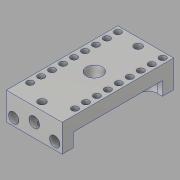
# Autodesk Inventor part: PocketNC_Vise_part2
Saved by Autodesk Inventor 2017 (Build 210142000, 142)
## iProperties
Created: 2018-06-05
Part Number: PocketNC_Vise_part2
Material: Aluminum 6061
Document SubType Name: Modeling
Designer: Jarrett
Density: 2.7 g/cm^3
Appearance: Aluminum - Flat
Author: Jarrett
Autodesk Inventor part; units mm, degrees
ref_plane "YZ Plane" through (0, 0, 0) normal (1, 0, 0) x (0, 1, 0)
ref_plane "XZ Plane" through (0, 0, 0) normal (0, 1, 0) x (-1, 0, 0)
ref_plane "XY Plane" through (0, 0, 0) normal (0, 0, 1) x (1, 0, 0)
sketch "Sketch1" plane through (0, 0, 0) normal (0, 1, 0) x (-1, 0, 0)
  line L0 (0, 0) -> (12.71, 0) construction
  line L1 (12.71, 25.41) -> (-12.71, 25.41)
  line L2 (-12.71, 25.41) -> (-12.71, -25.41)
  line L3 (-12.71, -25.41) -> (12.71, -25.41)
  line L4 (12.71, 25.41) -> (12.71, -25.41)
  dimension "d0" = 12.71
  dimension "d1" = 25.41
  dimension "d2" = 25.42
  dimension "d3" = 50.82
  constraints: 10 end point, 2 vertical, 1 horizontal, 1 perpendicular
  measures "d0" distance of L0.start L0.end
  measures "d1" distance of L0.end L1.start
  measures "d2" distance of L1.start L1.end
  measures "d3" distance of L1.end L2.end
extrude "Extrusion1" add sketch "Sketch1" along normal mid plane 12.6
sketch "Sketch2" plane through (0, -6.3, 0) normal (0, -1, 0) x (1, 0, 0)
  line L0 (12.71, 25.41) -> (12.71, 20.31) construction
  line L1 (12.71, 20.31) -> (6.26, 20.31)
  line L2 (12.71, -25.41) -> (12.71, -20.31) construction
  line L3 (12.71, -20.31) -> (6.26, -20.31)
  line L4 (6.26, -20.31) -> (6.26, 20.31)
  line L5 (12.71, 20.31) -> (12.71, -20.31)
  line L6 (12.71, 25.41) -> (12.71, -25.41) projected
  line L7 (0, 25.41) -> (0, -25.41)
  line L8 (-12.71, 20.31) -> (-6.26, 20.31)
  line L9 (-12.71, -20.31) -> (-6.26, -20.31)
  line L10 (-6.26, -20.31) -> (-6.26, 20.31)
  line L11 (-12.71, 20.31) -> (-12.71, -20.31)
  point P0 (0, 0)
  dimension "d6" = 5.1
  dimension "d7" = 6.45
  dimension "d8" = 5.1
  dimension "d9" = 6.45
  constraints: 22 end point, 4 symmetric about line, 2 perpendicular, 1 collinear, 1 vertical
  measures "d6" distance of L0.start L0.end
  measures "d7" distance of L0.end L1.end
  measures "d8" distance of L2.start L2.end
  measures "d9" distance of L2.end L3.end
extrude "Extrusion2" cut sketch "Sketch2" against normal blind 6.25
fillet "Fillet1" radius 4 4 edges at (6.26, -3.175, 20.31) (6.26, -3.175, -20.31) (-6.26, -3.175, -20.31) (-6.26, -3.175, 20.31)
sketch "Sketch3" plane through (0, 6.3, 0) normal (0, 1, 0) x (1, 0, 0)
  line L0 (-12.71, 25.41) -> (-12.71, 22.91) construction
  line L1 (-12.71, 22.91) -> (-10.21, 22.91) construction
  circle A0 centre (-10.21, 22.91) radius 1.5
  circle A1 centre (-10.21, -17.09) radius 1.5
  circle A2 centre (-10.21, -12.09) radius 1.5
  circle A3 centre (-10.21, -7.09) radius 1.5
  circle A4 centre (-10.21, -2.09) radius 1.5
  circle A5 centre (-10.21, 2.91) radius 1.5
  circle A6 centre (-10.21, 7.91) radius 1.5
  circle A7 centre (-10.21, 12.91) radius 1.5
  circle A8 centre (-10.21, 17.91) radius 1.5
  circle A9 centre (10.21, 22.91) radius 1.5
  circle A10 centre (10.21, -17.09) radius 1.5
  circle A11 centre (10.21, -12.09) radius 1.5
  circle A12 centre (10.21, -7.09) radius 1.5
  circle A13 centre (10.21, -2.09) radius 1.5
  circle A14 centre (10.21, 2.91) radius 1.5
  circle A15 centre (10.21, 7.91) radius 1.5
  circle A16 centre (10.21, 12.91) radius 1.5
  circle A17 centre (10.21, 17.91) radius 1.5
  circle A18 centre (0, 21.91) radius 1.75 construction
  line L2 (0, 0) -> (0, 21.91) construction
  line L3 (0, 0) -> (0, -21.91) construction
  circle A19 centre (0, -21.91) radius 1.75 construction
  circle A20 centre (0, -21.91) radius 1.5
  circle A21 centre (0, 21.91) radius 1.5
  line L4 (0, -21.91) -> (0, 1.95) construction
  circle A22 centre (0, 1.95) radius 2.2
  dimension "d13" = 2.5
  dimension "d15" = 3
  dimension "d25" = 3
  dimension "d26" = 3
  dimension "d27" = 3
  dimension "d28" = 3
  dimension "d29" = 3
  dimension "d30" = 3
  dimension "d31" = 3
  dimension "d32" = 3
  dimension "d33" = 5
  dimension "d35" = 3.5
  dimension "d36" = 21.91
  dimension "d38" = 21.91
  dimension "d39" = 3.5
  dimension "d40" = 3
  dimension "d41" = 3
  dimension "d42" = 23.86
  dimension "d43" = 4.4
  constraints: 23 centre point, 10 end point, 6 coincident, 1 perpendicular, 1 point on line, 1 vertical
  measures "d13" distance of L0.start L0.end
  measures "d15" diameter of A0
  measures "d25" diameter of A1
  measures "d26" diameter of A2
  measures "d27" diameter of A3
  measures "d28" diameter of A4
  measures "d29" diameter of A5
  measures "d30" diameter of A6
  measures "d31" diameter of A7
  measures "d32" diameter of A8
  measures "d33" distance of A5.centre A4.centre
  measures "d35" diameter of A18
  measures "d36" distance of L2.start L2.end
  measures "d38" distance of L2.start L3.end
  measures "d39" diameter of A19
  measures "d40" diameter of A20
  measures "d41" diameter of A21
  measures "d42" distance of L4.start L4.end
  measures "d43" diameter of A22
extrude "Extrusion3" cut sketch "Sketch3" against normal blind 15.775
sketch "Sketch4" plane through (0, 6.3, 0) normal (0, 1, 0) x (1, 0, 0)
  circle A0 centre (0, -21.91) radius 1.75
  circle A1 centre (0, 21.91) radius 1.75
  point P0 (0, 0)
  dimension "d46" = 3.5
  dimension "d47" = 3.5
  constraints: 2 centre point, 2 coincident
  measures "d46" diameter of A0
  measures "d47" diameter of A1
extrude "Extrusion4" cut sketch "Sketch4" against normal blind 4.6
sketch "Sketch5" plane through (0, 6.3, 0) normal (0, 1, 0) x (1, 0, 0)
  circle A0 centre (0, 1.95) radius 3.65
  point P0 (0, 0)
  dimension "d50" = 7.3
  constraints: 1 centre point, 1 coincident
  measures "d50" diameter of A0
extrude "Extrusion5" cut sketch "Sketch5" against normal blind 5.7
sketch "Sketch6" plane through (-12.71, 6.3, 25.41) normal (0, 0, 1) x (1, 0, 0)
  line L0 (25.42, -12.6) -> (22.07, -12.6) construction
  line L1 (22.07, -12.6) -> (22.07, -9.25) construction
  circle A0 centre (22.07, -9.25) radius 2.35
  line L2 (12.71, -0.1064) -> (12.71, -12.6)
  circle A1 centre (3.35, -9.25) radius 2.35
  circle A2 centre (12.71, -6.3) radius 2.425
  dimension "d53" = 3.35
  dimension "d54" = 3.35
  dimension "d55" = 4.7
  dimension "d56" = 4.85
  constraints: 6 end point, 3 centre point, 2 coincident, 1 horizontal, 1 perpendicular, 1 symmetric about line, 1 vertical, 1 other
  measures "d53" distance of L0.start L0.end
  measures "d54" distance of L0.end L1.end
  measures "d55" diameter of A0
  measures "d56" diameter of A2
extrude "Extrusion6" cut sketch "Sketch6" against normal blind 13.5
body "Solid1"
